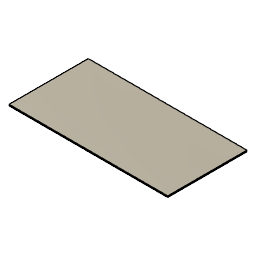
pannello_eps_1000x500x8mm (Autodesk Fusion 360 design; units mm, degrees)
Autodesk Fusion 360 part; units mm, degrees
sketch "Schizzo1" plane through (0, 0, 0) normal (0, 0, 1) x (1, 0, 0)
  line L0 (500, 250) -> (-500, 250)
  line L1 (-500, 250) -> (-500, -250)
  line L2 (-500, -250) -> (500, -250)
  line L3 (500, -250) -> (500, 250)
  line L4 (500, 250) -> (-500, -250) construction
  line L5 (-500, 250) -> (500, -250) construction
  dimension "d1" = 500
  dimension "d2" = 1000
  constraint horizontal L0
  constraint perpendicular L0 L1
  constraint parallel L0 L2
  constraint parallel L1 L3
  constraint coincident L4 origin
  constraint coincident L5 origin
  measures "d1" distance of L0.end L1.end
  measures "d2" distance of L0.start L0.end
extrude "Estrusione1" add sketch "Schizzo1" along normal blind 8
